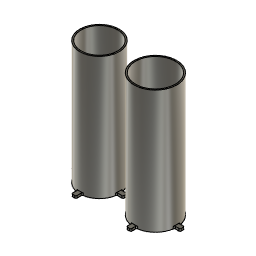
poc_4 (Autodesk Fusion 360 design; units mm, degrees)
Autodesk Fusion 360 part; units mm, degrees
sketch "Sketch1" plane through (0, 0, 0) normal (0, 0, 1) x (1, 0, 0)
  circle A0 centre (0, 0) radius 17.5
  dimension "d1" = 35
  constraint coincident A0.centre origin
  measures "d1" diameter of A0
extrude "Extrude1" add sketch "Sketch1" along normal blind 110 makes body 1
hole "Hole1" at (0, 0, 110) direction (0, 0, -1) diameter 32.6 depth 108 tip angle 180 bodies 1
fillet "Fillet1" radius 2 1 edges at (-15.1969, 5.8943, 2) on bodies 1
sketch "Sketch2" plane through (0, 0, 0) normal (0, 0, 1) x (1, 0, 0)
  circle A0 centre (50, 0) radius 19
  dimension "d9" = 38
  measures "d9" diameter of A0
extrude "Extrude2" add sketch "Sketch2" along normal blind 110 separate body makes body 2
hole "Hole2" at (50, 0, 110) direction (0, 0, -1) diameter 35.6 depth 108 tip angle 180 bodies 2
hole "Hole3" at (0, 0, 0) direction (0, 0, 1) diameter 19 depth 2 tip angle 180 bodies 1
sketch "Sketch5" plane through (0, 0, 0) normal (0, 0, -1) x (1, 0, 0)
  circle A0 centre (50, 0) radius 19
  line L0 (48, 24) -> (52, 24)
  line L1 (52, 24) -> (52, -24)
  line L2 (52, -24) -> (48, -24)
  line L3 (48, -24) -> (48, 24)
  line L4 (48, 24) -> (52, -24) construction
  line L5 (52, 24) -> (48, -24) construction
  point P0 (50, 0)
  dimension "d33" = 4
  dimension "d34" = 48
  constraint horizontal L0
  constraint perpendicular L0 L1
  constraint parallel L0 L2
  constraint parallel L1 L3
  constraint coincident L4 P0
  constraint coincident L5 P0
  constraint coincident P0 A0.centre
  measures "d33" distance of L1.end L2.end
  measures "d34" distance of L0.end L1.end
extrude "Extrude5" add sketch "Sketch5" against normal blind 2 contours A0 L0 L1 L3 | A0 L1 L2 L3 bodies 2
fillet "Fillet5" radius 1 8 edges at (52, -24, 1) (52, -18.8944, 1) (48, -24, 1) (48, -18.8944, 1) (52, 18.8944, 1) (52, 24, 1) (48, 24, 1) (48, 18.8944, 1) on bodies 2
pattern_circular "C-Pattern3" count 2 over 90 about axis through (50, 0, 0) along (0, 0, 1) of "Extrude5", "Fillet5"
sketch "Sketch6" plane through (0, 0, 0) normal (0, 0, -1) x (1, 0, 0)
  circle A0 centre (0, 0) radius 9.5
  circle A1 centre (0, 0) radius 17.5
  line L0 (-2, -23) -> (2, -23)
  line L1 (2, -23) -> (2, 23)
  line L2 (2, 23) -> (-2, 23)
  line L3 (-2, 23) -> (-2, -23)
  line L4 (-2, -23) -> (2, 23) construction
  line L5 (2, -23) -> (-2, 23) construction
  dimension "d41" = 4
  dimension "d42" = 46
  constraint horizontal L0
  constraint perpendicular L0 L1
  constraint parallel L0 L2
  constraint parallel L1 L3
  constraint coincident L4 A0.centre
  constraint coincident L5 A0.centre
  constraint coincident A0.centre A1.centre
  measures "d41" distance of L1.end L2.end
  measures "d42" distance of L0.end L1.end
extrude "Extrude6" add sketch "Sketch6" against normal blind 2 contours A1 L1 L2 L3 | A1 L0 L1 L3 bodies 1
fillet "Fillet6" radius 1 8 edges at (-2, -17.3853, 1) (-2, -23, 1) (2, -23, 1) (2, -17.3853, 1) (-2, 17.3853, 1) (-2, 23, 1) (2, 23, 1) (2, 17.3853, 1) on bodies 1
pattern_circular "C-Pattern4" count 2 over 90 about axis through (0, 0, 0) along (0, 0, 1) of "Extrude6", "Fillet6"
